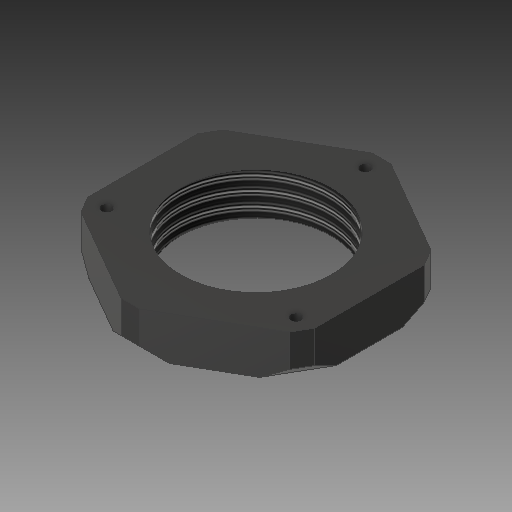
# Autodesk Inventor part: nut
Saved by Autodesk Inventor 2018 (Build 220112000, 112)
## iProperties
Created: 2019-04-16
Part Number: nut
Material: Generic
Document SubType Name: Modeling
Designer: ZEUSLAP
Density: 1 g/cm^3
Appearance: Default
Mass: 0.880848 g
Surface Area: 9.17254 cm^2
Volume: 0.880848 cm^3
Author: ZEUSLAP
Autodesk Inventor part; units mm, degrees
ref_plane "YZ Plane" through (0, 0, 0) normal (1, 0, 0) x (0, 1, 0)
ref_plane "XZ Plane" through (0, 0, 0) normal (0, 1, 0) x (-1, 0, 0)
ref_plane "XY Plane" through (0, 0, 0) normal (0, 0, 1) x (1, 0, 0)
sketch "Sketch1" plane through (0, 0, 0) normal (0, 1, 0) x (-1, 0, 0)
  line L0 (0, 0) -> (10.5, 0) construction
  line L1 (10.5, -6.0622) -> (0, -12.1244)
  line L2 (0, -12.1244) -> (-10.5, -6.0622)
  line L3 (-10.5, -6.0622) -> (-10.5, 6.0622)
  line L4 (-10.5, 6.0622) -> (0, 12.1244)
  line L5 (0, 12.1244) -> (10.5, 6.0622)
  line L6 (10.5, 6.0622) -> (10.5, -6.0622)
  circle A0 centre (0, 0) radius 7
  dimension "d0" = 10.5
  dimension "d1" = 14
  constraints: 14 end point, 2 coincident, 1 centre point, 1 horizontal, 1 midpoint, 13 other
  measures "d0" distance of L0.start L0.end
  measures "d1" diameter of A0
extrude "Extrusion1" add sketch "Sketch1" along normal blind 4
thread "Thread1" size "M14x1.25" class "6H" standard "ANSI Metric M Profile" full length
chamfer "Chamfer1" distance 1 angle 45 6 edges at (10.5, 2, 6.0622) (10.5, 2, -6.0622) (0, 2, -12.1244) (-10.5, 2, -6.0622) (-10.5, 2, 6.0622) (0, 2, 12.1244)
chamfer "Chamfer2" distance 1 angle 45 6 edges at (-10.067, 0, -5.8122) (0, 0, -11.6244) (-10.067, 0, 5.8122) (10.067, 0, -5.8122) (10.067, 0, 5.8122) (0, 0, 11.6244)
sketch "Sketch2" plane through (0, 4, 0) normal (0, 1, 0) x (1, 0, 0)
  circle A0 centre (0, 10.1244) radius 0.5
  line L0 (-0.866, 11.6244) -> (0.866, 11.6244) projected
  circle A1 centre (-8.7679, -5.0622) radius 0.5
  circle A2 centre (8.7679, -5.0622) radius 0.5
  point P0 (0, 0)
  dimension "d12" = 1
  dimension "d13" = 1.5
  dimension "d16" = 360
  constraints: 3 centre point, 7 other
  measures "d12" diameter of A0
  measures "d13" distance from line of L0 A0.centre
extrude "Extrusion2" cut sketch "Sketch2" against normal blind 2
sketch "Sketch3" plane through (0, 0, 0) normal (0, -1, 0) x (1, 0, 0)
  circle A0 centre (0, 0) radius 8.5
  dimension "d20" = 17
  constraints: 1 centre point, 1 coincident
  measures "d20" diameter of A0
extrude "Extrusion3" cut sketch "Sketch3" against normal blind 0.1
body "Solid1"
